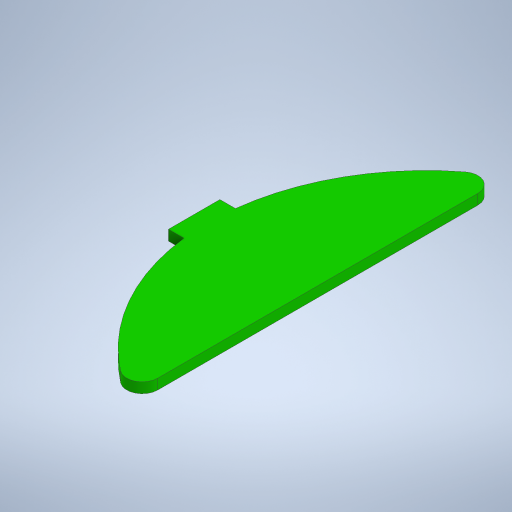
# Autodesk Inventor part: Test_PCB
Saved by Autodesk Inventor 2024 (Build 280153000, 153)
## iProperties
Created: 2025-01-20
Part Number: Test_PCB
Material: Générique
Document SubType Name: Modeling
Designer: malam
Density: 1 g/cm^3
Appearance: Par défaut
Author: malam
Autodesk Inventor part; units mm, degrees
ref_plane "YZ Plane" through (0, 0, 0) normal (1, 0, 0) x (0, 1, 0)
ref_plane "XZ Plane" through (0, 0, 0) normal (0, 1, 0) x (-1, 0, 0)
ref_plane "XY Plane" through (0, 0, 0) normal (0, 0, 1) x (1, 0, 0)
sketch "Esquisse1" plane through (0, 0, 0) normal (0, 1, 0) x (-1, 0, 0)
  line L0 (18.0036, -31.6819) -> (18.0036, -41.5796)
  line L1 (18.0036, 33.4181) -> (18.0036, -31.6819)
  line L2 (18.0036, 33.4181) -> (18.0036, 41.5796)
  arc A0 (18.0036, -41.5796) -> (18.0036, 41.5796) centre (0, 0) ccw
  line L3 (21.0036, 36.7285) -> (21.0036, 33.4181)
  line L4 (21.0036, 33.4181) -> (21.0036, -31.6819)
  line L5 (21.0036, -31.6819) -> (21.0036, -36.7285)
  arc A1 (21.0036, -36.7285) -> (21.0036, 36.7285) centre (0, 0) ccw
  line L6 (45.0333, 5) -> (42.0135, 5)
  line L7 (42.0135, 5) -> (42.0135, -5)
  line L8 (42.0135, -5) -> (45.0333, -5)
  line L9 (45.0333, -5) -> (45.0333, 5)
  line L10 (45.0333, 5) -> (42.0135, -5) construction
  line L11 (42.0135, 5) -> (45.0333, -5) construction
  line L12 (49.818, 0) -> (34.3139, 0) construction
  point P0 (0, 0)
  point P1 (43.5234, 0)
  dimension "d7" = 90.62
  dimension "d8" = 3
  dimension "d9" = 10
  constraints: 26 end point, 7 point on circle, 2 centre point, 2 horizontal, 2 midpoint, 2 parallel, 1 perpendicular, 1 vertical, 4 other
  measures "d7" diameter of A0
  measures "d8" radial gap between concentric circles of A0 A1
  measures "d9" distance of L7.end L6.end
extrude "Extrusion1" add sketch "Esquisse1" along normal blind 2 contours L8 A1 L6 L9 | L7 A1 | A1 L5 L4 L3 L7
fillet "Congé2" radius 3 2 edges at (-21.0036, 1, 36.7285) (-21.0036, 1, -36.7285)
